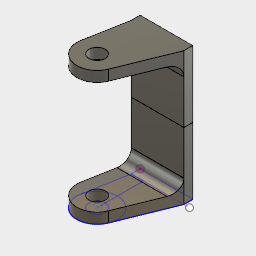
servo_bracket_ancle_2 (Autodesk Fusion 360 design; units mm, degrees)
Autodesk Fusion 360 part; units mm, degrees
sketch "スケッチ1" plane through (0, 0, 0) normal (0, 1, 0) x (1, 0, 0)
  line L0 (0, 0) -> (13, 0)
  line L1 (13, 0) -> (13, -2.2)
  line L2 (13, -2.2) -> (0, -2.2)
  line L3 (0, -2.2) -> (0, 0)
  line L4 (0, -2.2) -> (3, -2.2)
  line L5 (3, -2.2) -> (3, -13.6)
  line L6 (3, -2.2) -> (14.4, -2.2) construction
  circle A0 centre (3, -13.6) radius 5
  circle A1 centre (3, -13.6) radius 2
  line L7 (0, -2.2) -> (-1.9186, -12.7014)
  line L8 (13, -2.2) -> (7.6357, -15.4735)
  dimension "d1" = 2.2
  dimension "d2" = 13
  dimension "d3" = 3
  dimension "d4" = 90
  dimension "d5" = 11.4
  dimension "d6" = 10
  dimension "d7" = 4
  constraint horizontal L0
  constraint vertical L1
  constraint horizontal L2
  constraint vertical L3
  constraint horizontal L6
  constraint concentric A0 A1
  constraint coincident A0
  constraint tangent A0 L7
  constraint tangent A0 L8
  measures "d4" angle of L5 L6
  measures "d6" diameter of A0
  measures "d7" diameter of A1
extrude "押し出し1" add sketch "スケッチ1" along normal blind 2.6 contours L2 L4 L5 A0 L7 | L2 L5 A0 L8 | A0 makes body 1
extrude "押し出し2" add sketch "スケッチ1" along normal blind 16.425 contours L0 L1 L2 L3 L4 bodies 1
fillet "フィレット1" radius 3 1 edges at (6.5, 2.6, 2.2) on bodies 1
ref_plane "作業平面1" through (6.5, 16.425, 1.1) normal (0, 1, 0) x (0, 0, 1)
mirror "ミラー1" about plane through (6.5, 16.425, 1.1) normal (0, 1, 0) of bodies 1 makes body 2
